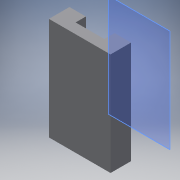
# Autodesk Inventor part: commutator_attachement_cable_cap
Saved by Autodesk Inventor 2016 (Build 200138000, 138)
## iProperties
Created: 2016-09-29
Part Number: commutator_attachement_cable_cap
Material: Generic
Document SubType Name: Modeling
Designer: ajar021
Density: 1 g/cm^3
Appearance: Default
Author: ajar021
Autodesk Inventor part; units mm, degrees
ref_plane "YZ Plane" through (0, 0, 0) normal (1, 0, 0) x (0, 1, 0)
ref_plane "XZ Plane" through (0, 0, 0) normal (0, 1, 0) x (-1, 0, 0)
ref_plane "XY Plane" through (0, 0, 0) normal (0, 0, 1) x (1, 0, 0)
sketch "Sketch1" plane through (0, 0, 0) normal (0, 0, 1) x (1, 0, 0)
  line L0 (-1.75, -10) -> (1.75, -10) projected
  line L1 (6, 10) -> (-6, 10) projected
  line L2 (-6, -10) -> (-6, 10) projected
  line L3 (6, 10) -> (6, -10) projected
  line L4 (6, -10) -> (1.75, -10) projected
  line L5 (-1.75, -10) -> (-6, -10) projected
  line L6 (0, 10) -> (-2.8, 10)
  line L7 (0, 10) -> (2.8, 10)
  line L8 (0, -10) -> (-2.8, -10)
  line L9 (0, -10) -> (2.8, -10)
  line L10 (-2.8, -10) -> (-2.8, 10)
  line L11 (2.8, -10) -> (2.8, 10)
  line L12 (2.8, 10) -> (6, 10)
  line L13 (2.8, 10) -> (6, 10)
  line L14 (6, -10) -> (6, 10)
  line L15 (6, -10) -> (2.8, -10)
  line L16 (-2.8, -10) -> (-6, -10)
  line L17 (-6, -10) -> (-6, 10)
  line L18 (-2.8, 10) -> (-6, 10)
  point P0 (0, 0)
  dimension "d0" = 2.8
  dimension "d1" = 2.8
  dimension "d2" = 2.8
  dimension "d3" = 2.8
  constraints: 26 end point, 6 collinear, 4 point on line, 2 midpoint, 1 perpendicular
  measures "d0" distance of L9.end L8.start
  measures "d1" distance of L8.end L8.start
  measures "d2" distance of L7.end L6.start
  measures "d3" distance of L6.end L6.start
extrude "Extrusion1" add sketch "Sketch1" along normal blind 2 contours L5 L2 L1 L10 | L11 L1 L3 L4
sketch "Sketch2" plane through (0, 0, 2) normal (0, 0, 1) x (1, 0, 0)
  line L0 (-6, 10) -> (-6, -10) projected
  line L1 (-6, -10) -> (-2.8, -10) projected
  line L2 (6, 10) -> (2.8, 10) projected
  line L3 (-6, 10) -> (6, 10)
  line L4 (6, -10) -> (6, 10) projected
  line L5 (6, 10) -> (6, -10)
  line L6 (6, -10) -> (-6, -10)
  line L7 (-6, 10) -> (-6, -10)
  point P0 (0, 0)
  constraints: 8 end point, 2 perpendicular, 1 collinear, 1 horizontal
extrude "Extrusion2" add sketch "Sketch2" along normal blind 2
equation "\"d0\" = d3"
equation "\"d1\" = d3"
equation "\"d2\" = d3"
body "Solid1"
